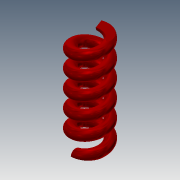
# Autodesk Inventor part: spring
Saved by Autodesk Inventor 2015 (Build 190159000, 159)
## iProperties
Created: 2021-04-19
Part Number: spring
Material: Stainless Steel, 440C
Document SubType Name: Modeling
Designer: Diptanshu Das
Density: 7.75 g/cm^3
Appearance: Semi-Polished(2)
Author: Diptanshu Das
Autodesk Inventor part; units mm, degrees
ref_plane "YZ Plane" through (0, 0, 0) normal (1, 0, 0) x (0, 1, 0)
ref_plane "XZ Plane" through (0, 0, 0) normal (0, 1, 0) x (-1, 0, 0)
ref_plane "XY Plane" through (0, 0, 0) normal (0, 0, 1) x (1, 0, 0)
sketch "Sketch1" plane through (0, 0, 0) normal (0, 0, 1) x (1, 0, 0)
  circle A0 centre (0, 0) radius 22.5
  dimension "d0" = 45
  constraints: 1 centre point, 1 coincident
  measures "d0" diameter of A0
extrude "Extrusion1" add sketch "Sketch1" along normal blind 100
sketch "Sketch2" plane through (0, 0, 0) normal (1, 0, 0) x (0, 1, 0)
  line L0 (22.5, 100) -> (-22.5, 100) projected
  line L1 (-22.5, 0) -> (22.5, 0) projected
  circle A0 centre (-17, 0) radius 4
  line L2 (0, 0) -> (0, 100) construction
  dimension "d3" = 100
  dimension "d4" = 8
  dimension "d5" = 17
  constraints: 2 end point, 1 centre point, 1 midpoint, 1 point on line
  measures "d3" distance between parallel lines of L1 L0
  measures "d4" diameter of A0
  measures "d5" distance of L2.start A0.centre
coil "Coil1" sketch "Sketch2" operation intersect axis through (0, 0, 0) along (0, 0, 1) pitch 25 turns 4 hand right
equation "\"d7\" = d3"
body "Solid1"
